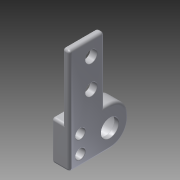
# Autodesk Inventor part: 13mmBearingBracketLeft
Saved by Autodesk Inventor 2015 (Build 190159000, 159)
## iProperties
Created: 2013-07-06
Part Number: 13mmBearingBracketLeft
Material: Generic
Document SubType Name: Modeling
Designer: mhgreen
Density: 1 g/cm^3
Appearance: Default
Author: mhgreen
Autodesk Inventor part; units mm, degrees
ref_plane "YZ Plane" through (0, 0, 0) normal (1, 0, 0) x (0, 1, 0)
ref_plane "XZ Plane" through (0, 0, 0) normal (0, 1, 0) x (-1, 0, 0)
ref_plane "XY Plane" through (0, 0, 0) normal (0, 0, 1) x (1, 0, 0)
sketch "Sketch1" plane through (0, 0, 0) normal (1, 0, 0) x (0, 1, 0)
  line L0 (27, 0) -> (27, -18)
  line L1 (0, 0) -> (0, -18)
  line L2 (27, -18) -> (0, -18)
  line L3 (0, 0) -> (27, 0)
  dimension "d2" = 18
  dimension "d11" = 27
  constraints: 8 end point, 1 parallel
  measures "d2" distance of L0.start L0.end
  measures "d11" distance of L1.start L0.start
sketch "Sketch2" plane through (0, 0, 0) normal (1, 0, 0) x (0, 1, 0)
  line L0 (0, 0) -> (16, 0)
  line L1 (16, 0) -> (16, 30)
  line L2 (16, 30) -> (0, 30)
  line L3 (0, 30) -> (0, 0)
  point P0 (7.5, 23)
  point P1 (8.5, 10)
  dimension "d8" = 30
  dimension "d9" = 7
  dimension "d10" = 10
  dimension "d66" = 16
  dimension "d71" = 7.5
  constraints: 8 end point, 2 parallel, 1 horizontal, 1 perpendicular, 1 vertical
  measures "d8" distance of L2.start L1.start
  measures "d9" distance from line of point (7.5, 23) L2
  measures "d10" distance from line of L0 point (8.5, 10)
  measures "d66" distance of L1.start point (0, 0)
  measures "d71" distance from line of L3 point (7.5, 23)
extrude "Extrusion1" add sketch "Sketch2" against normal blind 3.25
extrude "Extrusion2" add sketch "Sketch1" against normal blind 8.25
sketch "Sketch3" plane through (-3.25, 0, 0) normal (-1, 0, 0) x (0, 0, 1)
  line L0 (0, 16) -> (0, 0) projected
  line L1 (0, 0) -> (30, 0) projected
  line L2 (30, 0) -> (30, 16) projected
  point P0 (10, 10)
  point P1 (23, 10)
  dimension "d16" = 10
  dimension "d17" = 10
  dimension "d18" = 7
  dimension "d19" = 10
  measures "d16" distance from line of L1 point (10, 10)
  measures "d17" distance from line of L0 point (10, 10)
  measures "d18" distance from line of L2 point (23, 10)
  measures "d19" distance from line of L1 point (23, 10)
hole "Hole1" at (-3.25, 10, 10) at (-3.25, 10, 23) direction (1, 0, 0) diameter 5.3 end through all
sketch "Sketch4" plane through (-8.25, 0, 0) normal (-1, 0, 0) x (0, 0, 1)
  line L0 (0, 27) -> (-18, 27) projected
  line L1 (-18, 27) -> (-18, 0) projected
  point P0 (-9.5, 18.5)
  dimension "d27" = 8.5
  dimension "d28" = 8.5
  measures "d27" distance from line of L1 point (-9.5, 18.5)
  measures "d28" distance from line of L0 point (-9.5, 18.5)
hole "Hole2" at (-8.25, 18.5, -9.5) direction (1, 0, 0) diameter 13.06 depth 6.1
sketch "Sketch5" plane through (0, 0, 0) normal (1, 0, 0) x (0, 0, -1)
  line L0 (18, 0) -> (18, 27) projected
  line L1 (18, 27) -> (0, 27) projected
  point P0 (0, 0)
  point P1 (9.5, 18.5)
  dimension "d36" = 8.5
  dimension "d37" = 8.5
  measures "d36" distance from line of L0 point (9.5, 18.5)
  measures "d37" distance from line of L1 point (9.5, 18.5)
hole "Hole3" at (0, 18.5, -9.5) direction (-1, 0, 0) diameter 8 end through all
fillet "Fillet1" radius 8.5 2 edges at (-4.125, 27, -18) (-4.125, 27, 0)
sketch "Sketch7" plane through (-8.25, 0, 0) normal (-1, 0, 0) x (0, 0, 1)
  line L0 (-18, 18.5) -> (-18, 0) projected
  line L1 (-18, 0) -> (0, 0) projected
  line L2 (0, 0) -> (0, 18.5) projected
  point P0 (-5, 5)
  point P1 (-13, 5)
  dimension "d49" = 5
  dimension "d50" = 5
  dimension "d51" = 5
  dimension "d52" = 5
  measures "d49" distance from line of L0 point (-13, 5)
  measures "d50" distance from line of L2 point (-5, 5)
  measures "d51" distance from line of L1 point (-13, 5)
  measures "d52" distance from line of L1 point (-5, 5)
hole "Hole4" at (-8.25, 5, -5) at (-8.25, 5, -13) direction (1, 0, 0) diameter 4.4 end through all
fillet "Fillet3" radius 0.25 11 edges at (-8.25, 18.5, -16.03) (-2.15, 18.5, -5.5) (0, 18.5, -5.5) (-3.25, 10, 7.35) (-3.25, 10, 20.35) (0, 10, 7.35) (0, 10, 20.35) (-8.25, 5, -15.2) (-8.25, 5, -7.2) (0, 5, -7.2) (0, 5, -15.2)
fillet "Fillet4" radius 1.2 20 edges at (-8.25, 24.5104, -2.4896) (-8.25, 27, -9) (-8.25, 24.5104, -15.5104) (-8.25, 9.25, -18) (-8.25, 0, -9) (-8.25, 9.25, 0) (0, 24.5104, -2.4896) (0, 16, 15) (0, 8, 30) (0, 0, 6) (0, 9.25, -18) (0, 24.5104, -15.5104) (0, 27, -9) (-1.625, 0, 30) (-3.25, 0, 15) (-5.75, 0, 0) (-4.125, 0, -18) (-3.25, 16, 15) (-3.25, 8, 30) (-1.625, 16, 30)
body "Solid1"
